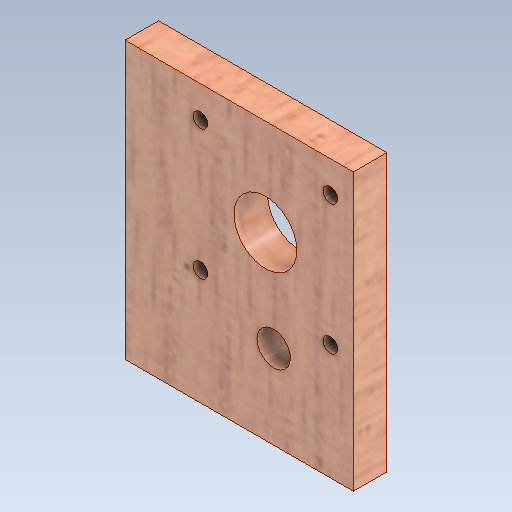
# Autodesk Inventor part: 0005-10-007Suport nema
Saved by Autodesk Inventor 2020 (Build 240168000, 168)
## iProperties
Created: 2020-12-18
Part Number: 0005-10-007Suport nema
Material: Generic
Document SubType Name: Modeling
Designer: Iulian Bors
Density: 1 g/cm^3
Appearance: White Oak - Natural Medium Gloss
Author: Iulian Bors
Subject: 007
Autodesk Inventor part; units mm, degrees
ref_plane "YZ Plane" through (0, 0, 0) normal (1, 0, 0) x (0, 1, 0)
ref_plane "XZ Plane" through (0, 0, 0) normal (0, 1, 0) x (-1, 0, 0)
ref_plane "XY Plane" through (0, 0, 0) normal (0, 0, 1) x (1, 0, 0)
sketch "Sketch1" plane through (0, 0, 0) normal (0, 0, 1) x (1, 0, 0)
  line L0 (-27.25, 33) -> (27.25, 33)
  line L1 (27.25, 33) -> (27.25, -33)
  line L2 (27.25, -33) -> (-27.25, -33)
  line L3 (-27.25, -33) -> (-27.25, 33)
  point P0 (0, 0)
  point P1 (0, 33)
  point P2 (-27.25, 0)
  dimension "d0" = 54.5
  dimension "d1" = 66
  constraints: 8 end point, 2 midpoint, 2 parallel, 1 horizontal, 1 horizontal alignment, 1 perpendicular, 1 vertical alignment
  measures "d0" distance of L0.start L0.end
  measures "d1" distance of L2.end L0.start
extrude "Extrusion1" add sketch "Sketch1" along normal blind 8
sketch "Sketch2" plane through (0, 0, 8) normal (0, 0, 1) x (1, 0, 0)
  circle A0 centre (6.25, 10) radius 7.5
  line L0 (27.25, 33) -> (-27.25, 33) projected
  line L1 (-27.25, 33) -> (-27.25, -33) projected
  line L2 (27.25, -33) -> (27.25, 33) projected
  line L3 (21.75, -5.5) -> (-9.25, -5.5) construction
  line L4 (-9.25, -5.5) -> (-9.25, 25.5) construction
  line L5 (-9.25, 25.5) -> (21.75, 25.5) construction
  line L6 (21.75, 25.5) -> (21.75, -5.5) construction
  line L7 (21.75, -5.5) -> (-9.25, 25.5) construction
  line L8 (-9.25, -5.5) -> (21.75, 25.5) construction
  circle A1 centre (-9.25, -5.5) radius 1.75
  circle A2 centre (-9.25, 25.5) radius 1.75
  circle A3 centre (21.75, 25.5) radius 1.75
  circle A4 centre (21.75, -5.5) radius 1.75
  point P0 (0, 33)
  point P1 (-27.25, 0)
  dimension "d17" = 15
  dimension "d19" = 21
  dimension "d20" = 23
  dimension "d22" = 31
  dimension "d23" = 3.5
  constraints: 12 end point, 5 centre point, 5 coincident, 5 midpoint, 3 equal radius, 2 parallel, 2 perpendicular, 1 horizontal
  measures "d17" diameter of A0
  measures "d19" distance from line of A0.centre L2
  measures "d20" distance from line of L0 A0.centre
  measures "d22" distance of L3.end L4.end
  measures "d23" diameter of A1
extrude "Extrusion2" cut sketch "Sketch2" against normal through all
sketch "Sketch4" plane through (0, 0, 8) normal (0, 0, 1) x (1, 0, 0)
  circle A0 centre (8.2191, -13) radius 4
  line L0 (-27.25, -33) -> (27.25, -33) projected
  line L1 (27.25, -33) -> (27.25, 33) projected
  point P0 (0, 0)
  dimension "d24" = 8
  dimension "d25" = 20
  dimension "d26" = 19.0309
  constraints: 1 centre point
  measures "d24" diameter of A0
  measures "d25" distance from line of L0 A0.centre
  measures "d26" distance from line of A0.centre L1
extrude "Extrusion4" cut sketch "Sketch4" against normal through all
body "Solid1"
